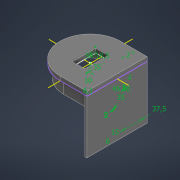
# Autodesk Inventor part: Celo
Saved by Autodesk Inventor 2022 (Build 260153000, 153)
## iProperties
Created: 2021-05-12
Part Number: Celo
Material: Generic
Document SubType Name: Modeling
Designer: jodyn
Density: 1 g/cm^3
Appearance: Gray
Author: jodyn
## iProperties of the stored document Celo_3DPrint.ipt
Created: 2021-05-12
Part Number: Celo_3DPrint
Material: Generic
Document SubType Name: Modeling
Designer: jodyn
Density: 1 g/cm^3
Appearance: Default
Author: jodyn
Autodesk Inventor part; units mm, degrees
ref_plane "YZ Plane" through (0, 0, 0) normal (1, 0, 0) x (0, 1, 0)
ref_plane "XZ Plane" through (0, 0, 0) normal (0, 1, 0) x (-1, 0, 0)
ref_plane "XY Plane" through (0, 0, 0) normal (0, 0, 1) x (1, 0, 0)
sketch "Sketch1" plane through (0, 0, 0) normal (0, 1, 0) x (-1, 0, 0)
  line L0 (62, 0) -> (-57, 0) projected
  line L1 (0, -63) -> (0, 63) projected
  line L2 (9.25, 17.5) -> (-9.25, 17.5)
  line L3 (-9.25, 17.5) -> (-9.25, -17.5)
  line L4 (-9.25, -17.5) -> (9.25, -17.5)
  line L5 (9.25, -17.5) -> (9.25, 17.5)
  circle A0 centre (0, 0) radius 33.5
  circle A1 centre (0, 0) radius 27
  line L6 (0, 45) -> (-40, 45)
  line L7 (-40, 45) -> (-40, -45)
  line L8 (-40, -45) -> (0, -45)
  arc A2 (0, -45) -> (0, 45) centre (0, 0) ccw
  line L9 (-13.1237, -34.8874) -> (-27, -34.8874)
  line L10 (-27, -34.8874) -> (-27, -24.7237)
  line L11 (-27, -24.7237) -> (-22.6051, -24.7237)
  line L12 (-13.1237, -30.8224) -> (-13.1237, -34.8874)
  circle A3 centre (-27.7874, 31.6695) radius 3.05
  circle A4 centre (-27.7874, 31.6695) radius 5
  line L13 (0, 40) -> (-35, 40)
  line L14 (-35, -40) -> (0, -40)
  arc A5 (0, -40) -> (0, 40) centre (0, 0) ccw
  line L15 (-35, -38) -> (0, -38)
  arc A6 (0, -38) -> (0, 38) centre (0, 0) ccw
  line L16 (0, 38) -> (-35, 38)
  line L17 (-35, -40) -> (-35, -38)
  line L18 (-35, 38) -> (-35, 40)
  dimension "d0" = 18.5
  dimension "d1" = 35
  dimension "d2" = 67
  dimension "d3" = 54
  dimension "d18" = 6.1
  dimension "d19" = 10
  dimension "d26" = 2
  constraints: 34 end point, 8 point on circle, 7 centre point, 7 parallel, 4 coincident, 4 point on line, 3 horizontal, 3 perpendicular, 2 midpoint, 1 collinear, 1 vertical, 5 other
  measures "d0" distance of L4.end L3.end
  measures "d1" distance of L3.end L2.end
  measures "d2" diameter of A0
  measures "d3" diameter of A1
  measures "d18" diameter of A3
  measures "d19" diameter of A4
  measures "d26" distance between parallel lines of L14 L15
extrude "Extrusion1" add sketch "Sketch1" along normal blind 5 contours A0 L1 A6 L0 | L0 A6 L1 A0 | A1 L1 L4 L5 L0 | L0 L5 L2 L1 A1 | A6 L1 A5 L0 | L0 A5 L1 A6 | A0 L0 L7 L6 L1 L13 L18 L16 | L1 L15 L17 L14 L8 L7 L0 A0 L11 L10 L9 L12 | L1 L2 L3 L0 A1 | A1 L0 L3 L4 L1 | A5 L1 A2 L0 | L0 A2 L1 A5 | L1 L14 L17 L15 | L16 L18 L13 L1 | L12 L9 L10 L11 A0 | A3 | A4
sketch "Sketch2" plane through (0, 5, 0) normal (0, 1, 0) x (1, 0, 0)
  line L0 (40, 45) -> (0, 45) projected
  arc A0 (0, 45) -> (0, -45) centre (0, 0) ccw projected
  line L1 (0, -45) -> (40, -45) projected
  line L2 (40, -45) -> (40, 45) projected
extrude "Extrusion2" add sketch "Sketch2" along normal blind 1
sketch "Sketch3" plane through (0, 5, 0) normal (0, -1, 0) x (1, 0, 0)
  line L0 (-9.25, -17.5) -> (9.25, -17.5) projected
  line L1 (9.25, -17.5) -> (9.25, 17.5) projected
  line L2 (9.25, 17.5) -> (-9.25, 17.5) projected
  line L3 (-9.25, 17.5) -> (-9.25, -17.5) projected
  point P0 (0, 0)
extrude "Extrusion3" cut sketch "Sketch3" against normal through all
extrude "Extrusion4" cut sketch "Sketch1" along normal blind 5 contours L12 L9 L10 L11 A0
sketch "Sketch4" plane through (0, 0, 0) normal (0, -1, 0) x (1, 0, 0)
  line L0 (40, -45) -> (0, -45) projected
  line L1 (40, 45) -> (40, -45) projected
  line L2 (0, 45) -> (40, 45) projected
  line L3 (40, -45) -> (37, -45)
  line L4 (37, -45) -> (37, 45)
  line L5 (37, 45) -> (40, 45)
  line L6 (40, 45) -> (40, -45)
  dimension "d14" = 3
  constraints: 8 end point, 2 parallel, 1 horizontal, 1 perpendicular, 1 point on line
  measures "d14" distance of L4.end L5.end
extrude "Extrusion5" add sketch "Sketch4" along normal blind 80
extrude "Extrusion6" add sketch "Sketch1" against normal blind 8 contours A4
extrude "Extrusion8" add sketch "Sketch1" against normal blind 20 contours A6 L1 A5 L0 | L0 A5 L1 A6 | L1 L14 L17 L15 | L16 L18 L13 L1
sketch "Sketch5" plane through (37, 0, -45) normal (-1, 0, 0) x (0, 0, 1)
  line L0 (0, -80) -> (90, -80) projected
  line L1 (37.5, -80) -> (52.5, -80)
  line L2 (52.5, -80) -> (52.5, -74)
  line L3 (52.5, -74) -> (37.5, -74)
  line L4 (37.5, -74) -> (37.5, -80)
  line L5 (0, 0) -> (0, -80) projected
  circle A0 centre (25.7628, -15.894) radius 1
  circle A1 centre (25.7628, -15.894) radius 2.5
  line L6 (25.7628, -7.1865) -> (25.7628, -27.0145) construction
  line L7 (25.7628, -15.894) -> (50.5115, -40.6428) construction
  line L8 (25.7628, -15.894) -> (60.7628, -15.894) construction
  circle A2 centre (50.5115, -40.6428) radius 1 construction
  circle A3 centre (50.5115, -40.6428) radius 2.5 construction
  circle A4 centre (50.5115, -40.6428) radius 1
  circle A5 centre (50.5115, -40.6428) radius 2.5
  dimension "d29" = 15
  dimension "d30" = 6
  dimension "d31" = 37.5
  dimension "d37" = 2
  dimension "d38" = 5
  dimension "d39" = 35
  dimension "d40" = 45
  dimension "d41" = 2
  dimension "d42" = 5
  constraints: 14 end point, 6 centre point, 5 coincident, 2 concentric, 2 horizontal, 2 parallel, 1 equal length, 1 perpendicular, 1 point on line, 1 vertical
  measures "d29" distance of L3.end L2.end
  measures "d30" distance of L2.end L1.end
  measures "d31" distance between parallel lines of L5 L4
  measures "d37" diameter of A0
  measures "d38" diameter of A1
  measures "d39" distance of L7.start L7.end
  measures "d40" angle of L7 L8
  measures "d41" diameter of A2
  measures "d42" diameter of A3
extrude "Extrusion9" add sketch "Sketch5" along normal blind 20 contours L4 L3 L2 L0
sketch "Sketch6" plane through (0, -80, 0) normal (0, -1, 0) x (1, 0, 0)
  circle A0 centre (27, 0) radius 1
  point P0 (0, 0)
  dimension "d34" = 2
  constraints: 1 centre point
  measures "d34" diameter of A0
extrude "Extrusion10" cut sketch "Sketch6" against normal blind 5
extrude "Extrusion11" add sketch "Sketch5" along normal blind 5 contours A1 | A5
body "Solid1"
